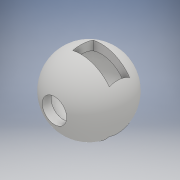
# Autodesk Inventor part: Деталь_4-19
Saved by Autodesk Inventor 2019 (Build 230136000, 136)
## iProperties
Created: 2020-04-05
Part Number: Деталь_4-19
Material: Типовые
Document SubType Name: Modeling
Designer: Diana
Density: 1 g/cm^3
Appearance: По умолчанию
Author: Diana
Autodesk Inventor part; units mm, degrees
ref_plane "YZ Plane" through (0, 0, 0) normal (1, 0, 0) x (0, 1, 0)
ref_plane "XZ Plane" through (0, 0, 0) normal (0, 1, 0) x (-1, 0, 0)
ref_plane "XY Plane" through (0, 0, 0) normal (0, 0, 1) x (1, 0, 0)
sketch "Эскиз1" plane through (0, 0, 0) normal (0, 0, 1) x (1, 0, 0)
  arc A0 (45, 0) -> (-45, 0) centre (0, 0) ccw
  arc A1 (35, 0) -> (-35, 0) centre (0, 0) ccw
  line L0 (-45, 0) -> (-35, 0)
  line L1 (35, 0) -> (45, 0)
  line L2 (-63, 0) -> (63, 0) projected
  dimension "d0" = 45
  dimension "d1" = 35
  constraints: 4 end point, 4 point on circle, 3 coincident, 2 centre point, 2 horizontal, 1 other
  measures "d0" radius of A0
  measures "d1" radius of A1
revolve "Вращение1" add sketch "Эскиз1" angle 360 about axis through (-10, 0, 0) along (1, 0, 0) contours L1 A1 L0 A0
sketch "Эскиз2" plane through (0, 0, 0) normal (0, 0, 1) x (1, 0, 0)
  circle A0 centre (0, 0) radius 15
  dimension "d3" = 30
  constraints: 1 centre point, 1 coincident
  measures "d3" diameter of A0
extrude "Выдавливание1" cut sketch "Эскиз2" along normal through all
sketch "Эскиз3" plane through (0, 0, 0) normal (0, 1, 0) x (-1, 0, 0)
  line L0 (-35, -15) -> (10, -15)
  line L1 (10, -15) -> (10, 10)
  line L2 (10, 10) -> (-35, 10)
  line L3 (-35, 10) -> (-35, -15)
  point P0 (0, 0)
  dimension "d6" = 10
  dimension "d7" = 45
  dimension "d8" = 10
  dimension "d9" = 25
  constraints: 8 end point, 2 parallel, 1 horizontal, 1 perpendicular
  measures "d6" distance from line of L1 point (0, 0)
  measures "d7" distance between parallel lines of L3 L1
  measures "d8" distance from line of point (0, 0) L2
  measures "d9" distance between parallel lines of L2 L0
extrude "Выдавливание2" cut sketch "Эскиз3" along normal through all both and the other way through all
